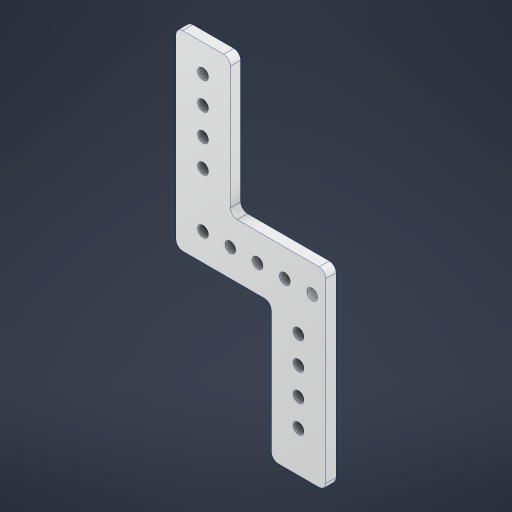
# Autodesk Inventor part: DVBS_007_Z-bracket1
Saved by Autodesk Inventor 2024 (Build 280153000, 153)
## iProperties
Created: 2024-07-29
Part Number: DVBS_007_Z-bracket1
Material: Aluminum 6061
Document SubType Name: Modeling
Designer: sarav
Density: 2.7 g/cm^3
Appearance: Aluminum - Flat
Author: sarav
Autodesk Inventor part; units mm, degrees
ref_plane "YZ Plane" through (0, 0, 0) normal (1, 0, 0) x (0, 1, 0)
ref_plane "XZ Plane" through (0, 0, 0) normal (0, 1, 0) x (-1, 0, 0)
ref_plane "XY Plane" through (0, 0, 0) normal (0, 0, 1) x (1, 0, 0)
sketch "Sketch1" plane through (0, 0, 0) normal (0, 0, 1) x (1, 0, 0)
  line L0 (12.7725, 14.853) -> (12.7725, 37.078)
  line L1 (9.5975, 40.253) -> (-28.5025, 40.253)
  line L2 (-15.8025, 14.853) -> (-53.9025, 14.853)
  line L3 (-57.0775, 18.028) -> (-57.0775, 40.253)
  line L4 (-31.6775, 43.428) -> (-31.6775, 100.578)
  line L5 (-34.8525, 103.753) -> (-53.9025, 103.753)
  line L6 (-57.0775, 100.578) -> (-57.0775, 40.253)
  line L7 (-57.0775, 40.253) -> (-31.6775, 40.253)
  line L8 (-12.6275, 14.853) -> (12.7725, 14.853)
  line L9 (12.7725, 14.853) -> (12.7725, -45.472)
  line L10 (9.5975, -48.647) -> (-9.4525, -48.647)
  line L11 (-12.6275, -45.472) -> (-12.6275, 11.678)
  arc A0 (-53.9025, 103.753) -> (-57.0775, 100.578) centre (-53.9025, 100.578) ccw
  arc A1 (-31.6775, 100.578) -> (-34.8525, 103.753) centre (-34.8525, 100.578) ccw
  arc A2 (-57.0775, 18.028) -> (-53.9025, 14.853) centre (-53.9025, 18.028) ccw
  arc A3 (-31.6775, 43.428) -> (-28.5025, 40.253) centre (-28.5025, 43.428) ccw
  arc A4 (-12.6275, -45.472) -> (-9.4525, -48.647) centre (-9.4525, -45.472) ccw
  arc A5 (9.5975, -48.647) -> (12.7725, -45.472) centre (9.5975, -45.472) ccw
  arc A6 (12.7725, 37.078) -> (9.5975, 40.253) centre (9.5975, 37.078) ccw
  arc A7 (-12.6275, 11.678) -> (-15.8025, 14.853) centre (-15.8025, 11.678) ccw
  point P0 (12.7725, 40.253)
  point P1 (-57.0775, 14.853)
  point P2 (-31.6775, 103.753)
  point P3 (-57.0775, 103.753)
  point P4 (12.7725, -48.647)
  point P5 (-12.6275, -48.647)
  point P6 (12.7725, 14.853)
  dimension "d7" = 25.4
  dimension "d15" = 25.4
  dimension "d17" = 44.45
  dimension "d18" = 44.45
  dimension "d19" = 25.4
  dimension "d20" = 63.5
  dimension "d21" = 25.4
  dimension "d58" = 63.5
  dimension "d59" = 3.175
  constraints: 24 end point, 17 point on line, 16 point on circle, 16 tangent, 8 centre point, 7 equal radius, 5 horizontal, 3 perpendicular, 3 vertical, 2 parallel
  measures "d7" distance of L8.start L0.start
  measures "d15" distance of L0.start point (12.772, 40.253)
  measures "d17" distance of point (12.772, 40.253) L7.end
  measures "d18" distance of L8.start point (-57.078, 14.853)
  measures "d19" distance of point (-57.078, 14.853) L3.end
  measures "d20" distance of L7.end point (-31.678, 103.753)
  measures "d21" distance of point (-31.678, 103.753) point (-57.078, 103.753)
  measures "d58" distance of L8.end point (12.772, -48.647)
  measures "d59" radius of A0
extrude "Extrusion1" add sketch "Sketch1" along normal blind 4.7625
sketch "Sketch2" plane through (0, 0, 4.7625) normal (0, 0, 1) x (1, 0, 0)
  line L0 (-57.0775, 100.578) -> (-57.0775, 18.028) projected
  line L1 (-53.9025, 14.853) -> (-15.8025, 14.853) projected
  line L2 (9.5975, 40.253) -> (-28.5025, 40.253) projected
  line L3 (-31.6775, 43.428) -> (-31.6775, 100.578) projected
  line L4 (-34.8525, 103.753) -> (-53.9025, 103.753) projected
  line L5 (-12.6275, 14.853) -> (12.7725, 14.853) construction
  circle A0 centre (0.0725, 8.4903) radius 2.5019
  line L6 (0.0725, 14.853) -> (0.0725, 10.9922) construction
  circle A1 centre (0.0725, -16.9097) radius 2.5019
  circle A2 centre (0.0725, -4.2097) radius 2.5019
  line L7 (0.0725, 5.9884) -> (0.0725, -1.7078) construction
  line L8 (0.0725, -6.7116) -> (0.0725, -14.4078) construction
  circle A3 centre (0.0725, -29.6097) radius 2.5019
  line L9 (0.0725, -19.4116) -> (0.0725, -27.1078) construction
  line L10 (-57.0775, 103.753) -> (-57.0775, 14.853) projected
  line L11 (12.7725, 14.853) -> (-57.0775, 14.853) construction
  line L12 (-57.0775, 14.853) -> (-57.0775, 40.253)
  line L13 (-57.0775, 40.253) -> (12.7725, 40.253) construction
  line L14 (12.7725, 40.253) -> (12.7725, 14.853)
  line L15 (-57.0775, 27.553) -> (12.7725, 27.553) construction
  circle A4 centre (6.4098, 27.553) radius 2.5019
  line L16 (8.9117, 27.553) -> (12.7725, 27.553)
  circle A5 centre (-6.2902, 27.553) radius 2.5019
  line L17 (-69.7775, 27.553) -> (0.0725, 27.553) construction
  circle A6 centre (-18.9902, 27.553) radius 2.5019
  line L18 (-82.4775, 27.553) -> (-12.6275, 27.553) construction
  circle A7 centre (-31.6902, 27.553) radius 2.5019
  line L19 (-95.1775, 27.553) -> (-25.3275, 27.553) construction
  circle A8 centre (-44.3902, 27.553) radius 2.5019
  line L20 (-107.8775, 27.553) -> (-38.0275, 27.553) construction
  line L21 (-44.3902, 40.253) -> (-44.3775, 101.2638) construction
  circle A9 centre (-44.3876, 52.9657) radius 2.5019
  line L22 (-44.3881, 50.4638) -> (-44.3902, 40.253)
  circle A10 centre (-44.3849, 65.6657) radius 2.5019
  circle A11 centre (-44.3823, 78.3657) radius 2.5019
  circle A12 centre (-44.3796, 91.0657) radius 2.5019
  line L23 (-12.6275, 11.678) -> (-12.6275, -45.472) projected
  line L24 (-9.4525, -48.647) -> (9.5975, -48.647) projected
  arc A13 (-31.6775, 43.428) -> (-28.5025, 40.253) centre (-28.5025, 43.428) ccw projected
  arc A14 (-31.6775, 100.578) -> (-34.8525, 103.753) centre (-34.8525, 100.578) ccw projected
  arc A15 (-53.9025, 103.753) -> (-57.0775, 100.578) centre (-53.9025, 100.578) ccw projected
  arc A16 (-57.0775, 18.028) -> (-53.9025, 14.853) centre (-53.9025, 18.028) ccw projected
  arc A17 (-12.6275, 11.678) -> (-15.8025, 14.853) centre (-15.8025, 11.678) ccw projected
  arc A18 (-12.6275, -45.472) -> (-9.4525, -48.647) centre (-9.4525, -45.472) ccw projected
  arc A19 (9.5975, -48.647) -> (12.7725, -45.472) centre (9.5975, -45.472) ccw projected
  line L25 (12.7725, -45.472) -> (12.7725, 37.078) projected
  arc A20 (12.7725, 37.078) -> (9.5975, 40.253) centre (9.5975, 37.078) ccw projected
  point P0 (0, 0)
  point P1 (-3.7883, 27.553)
  point P2 (-16.4883, 27.553)
  point P3 (-29.1883, 27.553)
  point P4 (-41.8883, 27.553)
  point P5 (-44.3854, 63.1638)
  point P6 (-44.3828, 75.8638)
  point P7 (-44.3801, 88.5638)
  dimension "d34" = 5.0038
  dimension "d38" = 5.0038
  dimension "d47" = 5.0038
  dimension "d26" = 5.0038
  dimension "d29" = 3.8608
  dimension "d30" = 5.0038
  dimension "d31" = 5.0038
  dimension "d32" = 7.6962
  dimension "d33" = 7.6962
  dimension "d35" = 7.6962
  dimension "d39" = 3.8608
  dimension "d42" = 12.7
  dimension "d48" = 10.2108
  dimension "d51" = 12.7
  constraints: 34 end point, 22 point on line, 6 horizontal, 6 point on circle, 5 horizontal alignment, 3 centre point, 3 collinear, 3 midpoint, 3 vertical, 2 parallel, 1 perpendicular, 1 vertical alignment, 56 other
  measures "d26" diameter of A0
  measures "d29" distance of L6.start L6.end
  measures "d30" diameter of A1
  measures "d31" diameter of A2
  measures "d32" distance of L7.start L7.end
  measures "d33" distance of L8.start L8.end
  measures "d35" distance of L9.start L9.end
  measures "d39" distance of L16.start L15.end
  measures "d42" distance of point (6.41, 27.553) point (-6.29, 27.553)
  measures "d48" distance of L22.start L21.start
  measures "d51" distance of point (-44.388, 52.966) point (-44.385, 65.666)
extrude "Extrusion2" cut sketch "Sketch2" against normal through all contours A4 | A0 | A1 | A2 | A3 | A5 | A6 | A7 | A8 | A9 | A10 | A11 | A12
body "Solid1"
